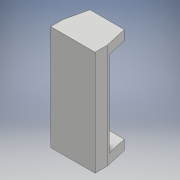
# Autodesk Inventor part: Part2
Saved by Autodesk Inventor 2017.3 (Build 213256000, 256)
## iProperties
Part Number: Part2
Material: 一般
Document SubType Name: Modeling
Designer: sktom
Density: 1 g/cm^3
Appearance: 既定
Author: sktom
Autodesk Inventor part; units mm, degrees
ref_plane "YZ Plane" through (0, 0, 0) normal (1, 0, 0) x (0, 1, 0)
ref_plane "XZ Plane" through (0, 0, 0) normal (0, 1, 0) x (-1, 0, 0)
ref_plane "XY Plane" through (0, 0, 0) normal (0, 0, 1) x (1, 0, 0)
sketch "スケッチ1" plane through (0, 0, 0) normal (0, 0, 1) x (1, 0, 0)
  line L0 (-9.05, -7) -> (9.05, -7)
  line L1 (9.05, -7) -> (9.05, 7)
  line L2 (9.05, 7) -> (-9.05, 7)
  line L3 (-9.05, 7) -> (-9.05, -7)
  line L4 (-9.05, -7) -> (9.05, 7) construction
  line L5 (9.05, -7) -> (-9.05, 7) construction
  point P0 (0, 0)
  dimension "d1" = 14
  dimension "d2" = 18.1
  constraints: 12 end point, 2 midpoint, 2 parallel, 1 horizontal, 1 perpendicular
  measures "d1" distance of L0.end L1.end
  measures "d2" distance of L0.start L0.end
extrude "押し出し1" add sketch "スケッチ1" along normal blind 42.8
sketch "スケッチ2" plane through (0, 0, 42.8) normal (0, 0, 1) x (1, 0, 0)
  line L0 (-9.05, 7) -> (-9.05, -7) projected
  line L1 (-9.05, 7) -> (-7, 7)
  line L2 (-7, 7) -> (-9.05, -2)
  line L3 (9.05, 7) -> (-9.05, 7) projected
  line L4 (-9.05, 7) -> (-9.05, -2)
  line L5 (9.05, -7) -> (9.05, 7) projected
  line L6 (9.05, 7) -> (9.05, -2)
  line L7 (9.05, -2) -> (7, 7)
  line L8 (7, 7) -> (9.05, 7)
  line L9 (-9.05, -7) -> (9.05, -7) projected
  point P0 (0, 0)
  dimension "d5" = 14
  dimension "d6" = 5
  constraints: 12 end point, 3 point on line, 2 perpendicular, 1 equal length, 1 horizontal, 1 horizontal alignment
  measures "d5" distance of L7.end L1.end
  measures "d6" distance from line of L9 L6.end
extrude "押し出し2" cut sketch "スケッチ2" against normal through all contours L1 L2 L0 | L3 L5 L7
sketch "スケッチ3" plane through (-7, 7, 0) normal (0, 1, 0) x (1, 0, 0)
  line L0 (-2.05, 0) -> (-2.05, -42.8) projected
  line L1 (16.05, 0) -> (16.05, -42.8) projected
  line L2 (-2.05, -38.8) -> (16.05, -38.8)
  line L3 (16.05, -38.8) -> (16.05, -4)
  line L4 (16.05, -4) -> (-2.05, -4)
  line L5 (-2.05, -4) -> (-2.05, -38.8)
  line L6 (14, 0) -> (0, 0) projected
  line L7 (14, -42.8) -> (0, -42.8) projected
  point P0 (7, 0)
  dimension "d9" = 4
  dimension "d10" = 4
  constraints: 8 end point, 2 parallel, 2 point on line, 1 horizontal, 1 perpendicular
  measures "d9" distance between parallel lines of L6 L4
  measures "d10" distance between parallel lines of L7 L2
extrude "押し出し3" cut sketch "スケッチ3" against normal blind 8
sketch "スケッチ4" plane through (-7, 7, 4) normal (0, 0, 1) x (1, 0, 0)
  circle A0 centre (7, -4.45) radius 8.25
  line L0 (-2.05, -14) -> (16.05, -14) projected
  point P0 (7, -7)
  dimension "d13" = 16.5
  dimension "d14" = 17.8
  constraints: 1 centre point, 1 vertical alignment
  measures "d13" diameter of A0
extrude "押し出し4" cut sketch "スケッチ4" along normal up to surface (34.8 mm away)
sketch "スケッチ5" plane through (-7, 7, 0) normal (0, 1, 0) x (1, 0, 0)
  line L0 (2.1, -3) -> (11.9, -3)
  line L1 (11.9, -3) -> (11.9, -1)
  line L2 (11.9, -1) -> (2.1, -1)
  line L3 (2.1, -1) -> (2.1, -3)
  line L4 (2.1, -3) -> (11.9, -1) construction
  line L5 (11.9, -3) -> (2.1, -1) construction
  line L6 (14, -4) -> (14, 0) projected
  line L7 (14, 0) -> (0, 0) projected
  point P0 (7, 0)
  point P1 (7, -2)
  point P2 (7, -2)
  point P3 (14, -2)
  point P4 (7, -2)
  point P5 (7, 0)
  dimension "d17" = 2
  dimension "d18" = 9.8
  constraints: 12 end point, 6 midpoint, 2 parallel, 1 horizontal, 1 horizontal alignment, 1 perpendicular, 1 vertical alignment
  measures "d17" distance of L0.end L1.end
  measures "d18" distance of L1.end L2.end
extrude "押し出し5" cut sketch "スケッチ5" against normal blind 13
